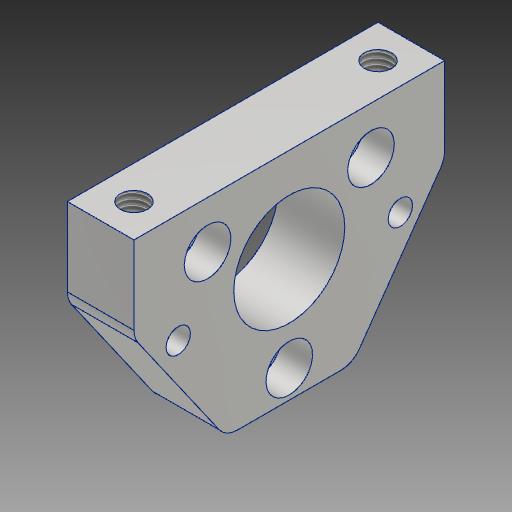
# Autodesk Inventor part: Motorhalter
Saved by Autodesk Inventor 2019.4 (Build 234330000, 330)
## iProperties
Part Number: Motorhalter
Material: Aluminium 6061
Document SubType Name: Modeling
Designer: rYan
Mass: 5.26955 g
Surface Area: 17.5753 cm^2
Volume: 1.95168 cm^3
Density: 2.7 g/cm^3
Appearance: Aluminium - flach
Author: rYan
Autodesk Inventor part; units mm, degrees
ref_plane "YZ Plane" through (0, 0, 0) normal (1, 0, 0) x (0, 1, 0)
ref_plane "XZ Plane" through (0, 0, 0) normal (0, 1, 0) x (-1, 0, 0)
ref_plane "XY Plane" through (0, 0, 0) normal (0, 0, 1) x (1, 0, 0)
sketch "Skizze1" plane through (0, 0, 0) normal (1, 0, 0) x (0, 1, 0)
  arc A0 (-6.9821, 8.5) -> (6.9821, 8.5) centre (0, 0) ccw construction
  line L0 (14, 8.5) -> (-14, 8.5)
  line L1 (-14, 8.5) -> (-14, 0.8162)
  line L2 (0, 12.4) -> (0, -14.9) projected
  circle A1 centre (0, 0) radius 5
  line L3 (14, 0.8162) -> (14, 8.5)
  line L4 (-14, 0.8162) -> (-5.7262, -11)
  line L5 (-5.7262, -11) -> (5.7262, -11)
  line L6 (5.7262, -11) -> (14, 0.8162)
  circle A2 centre (10.009, -1.351) radius 1.1
  circle A3 centre (-10.009, -1.351) radius 1.1
  dimension "d0" = 22
  dimension "d2" = 10
  dimension "d19" = 8.5
  dimension "d39" = 14
  dimension "d50" = 2.2
  dimension "d57" = 10.009
  dimension "d58" = 1.351
  dimension "d59" = 35
  constraints: 12 end point, 4 centre point, 2 coincident, 2 horizontal, 2 point on circle, 2 point on line, 2 tangent, 3 other
  measures "d0" diameter of A0
  measures "d2" diameter of A1
  measures "d19" distance from line of point (0, 0) L0
  measures "d39" distance between parallel lines of L1 L2
  measures "d50" diameter of A2
  measures "d57" horizontal distance of A2.centre point (0, 0)
  measures "d58" vertical distance of point (0, 0) A2.centre
  measures "d59" angle of L4 L1
extrude "Extrusion1" add sketch "Skizze1" along normal mid plane 6 contours L3 L6 L5 L2 A1 L0 | L2 A1 L5 L4 L1 L0
sketch "Skizze2" plane through (3, 0, 0) normal (1, 0, 0) x (0, 0, -1)
  circle A0 centre (0, 0) radius 8.5 construction
  line L0 (0, 0) -> (8.5, 0) construction
  line L1 (-12.4, 0) -> (14.9, 0) projected
  dimension "d6" = 17
  constraints: 2 end point, 1 coincident, 1 horizontal alignment, 1 point on line, 2 other
hole "Bohrung1" at (3, 0, -8.5) direction (-1, 0, 0) diameter 2.1 end through all counterbore diameter 4.2 counterbore depth 2.8
pattern_circular "Runde Anordnung1" count 3 over 360 about axis through (0, 0, 0) along (1, 0, 0) of "Bohrung1"
sketch "Skizze3" plane through (-3, -14, 8.5) normal (0, 0, 1) x (1, 0, 0)
  line L0 (0, 0) -> (6, 0) projected
  line L1 (6, 28) -> (6, 0) projected
  line L2 (0, 0) -> (0, 28) projected
  line L3 (0, 0) -> (6, 0) construction
  line L4 (3, 0) -> (3, 24.0467) construction
  line L5 (6, 28) -> (0, 28) projected
  line L6 (-1.2, 14) -> (7.2, 14) projected
  point P0 (3, 14)
  point P1 (3, 3)
  point P2 (3, 25)
  dimension "d44" = 11
  constraints: 2 end point, 2 point on line, 1 midpoint, 1 symmetric about line
  measures "d44" distance of point (3, 3) point (3, 14)
hole "Bohrung2" at (0, -11, 8.5) at (0, 11, 8.5) direction (0, 0, -1) diameter 2.459 depth 7 tip angle 118 thread size "M3x0.5" class "6H" standard "ISO Metric profile"
sketch "Skizze5" plane through (3, 0, 0) normal (1, 0, 0) x (0, 0, -1)
  circle A0 centre (0, 0) radius 6.5
  dimension "d41" = 13
  constraints: 1 centre point, 1 coincident
  measures "d41" diameter of A0
extrude "Extrusion2" [suppressed]
chamfer "Fase1" [suppressed]
fillet "Rundung2" radius 2 4 edges at (0, -5.7262, -11) (0, 5.7262, -11) (0, -14, 0.8162) (0, 14, 0.8162)
fillet "Rundung1" [suppressed]
